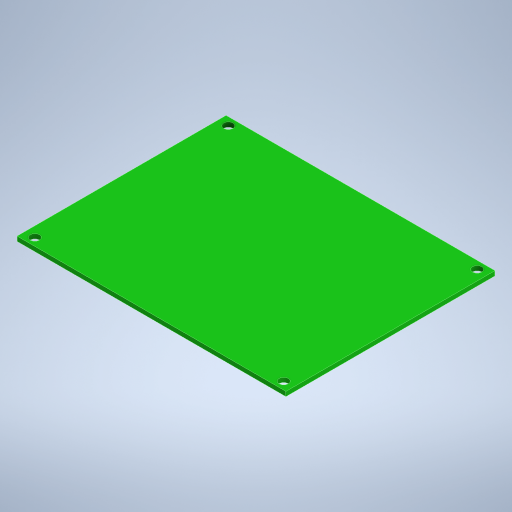
# Autodesk Inventor part: PCB
Saved by Autodesk Inventor 2024 (Build 280153000, 153)
## iProperties
Created: 2023-10-18
Part Number: PCB
Material: Generic
Document SubType Name: Modeling
Designer: CJ110
Density: 1 g/cm^3
Appearance: Default
Author: CJ110
Autodesk Inventor part; units mm, degrees
ref_plane "YZ Plane" through (0, 0, 0) normal (1, 0, 0) x (0, 1, 0)
ref_plane "XZ Plane" through (0, 0, 0) normal (0, 1, 0) x (-1, 0, 0)
ref_plane "XY Plane" through (0, 0, 0) normal (0, 0, 1) x (1, 0, 0)
sketch "Sketch1" plane through (0, 0, 0) normal (0, 1, 0) x (-1, 0, 0)
  line L0 (0, 0) -> (90.17, 0)
  line L1 (90.17, 0) -> (90.17, 70.104)
  line L2 (90.17, 70.104) -> (0, 70.104)
  line L3 (0, 70.104) -> (0, 0)
  dimension "PCB_Length" = 90.17
  dimension "PCB_Width" = 70.104
  constraints: 8 end point, 2 parallel, 1 horizontal, 1 perpendicular
  measures "PCB_Length" distance of L2.end L1.end
  measures "PCB_Width" distance of L0.end L1.end
extrude "Extrusion1" add sketch "Sketch1" along normal blind 1.524
sketch "Sketch2" plane through (0, 1.524, 0) normal (0, 1, 0) x (1, 0, 0)
  circle A0 centre (-3.3655, -2.6035) radius 1.5875
  circle A1 centre (-86.8045, -2.6035) radius 1.5875
  circle A2 centre (-86.8045, -67.5005) radius 1.5875
  circle A3 centre (-3.3655, -67.5005) radius 1.5875
  line L0 (-90.17, -70.104) -> (0, -70.104) projected
  line L1 (0, -70.104) -> (0, 0) projected
  line L2 (0, 0) -> (-90.17, 0) projected
  line L3 (-90.17, 0) -> (-90.17, -70.104) projected
  point P0 (-3.3655, -69.088)
  point P1 (-1.778, -67.5005)
  point P2 (-3.3655, -1.016)
  point P3 (-1.778, -2.6035)
  point P4 (-86.8045, -1.016)
  point P5 (-88.392, -2.6035)
  point P6 (-86.8045, -69.088)
  point P7 (-88.392, -67.5005)
  dimension "d4" = 3.175
  dimension "d5" = 1.016
  dimension "d6" = 1.778
  dimension "d7" = 1.016
  dimension "d8" = 1.778
  dimension "d9" = 1.016
  dimension "d10" = 1.778
  dimension "d11" = 1.016
  dimension "d12" = 1.778
  constraints: 8 point on circle, 4 centre point, 4 horizontal alignment, 4 vertical alignment, 3 equal radius
  measures "d4" diameter of A3
  measures "d5" distance from line of L0 A3.start
  measures "d6" distance from line of L1 A3.end
  measures "d7" distance from line of L2 A0.start
  measures "d8" distance from line of L1 A0.end
  measures "d9" distance from line of L0 A2.start
  measures "d10" distance from line of L3 A2.end
  measures "d11" distance from line of L2 A1.start
  measures "d12" distance from line of L3 A1.end
extrude "Extrusion2" cut sketch "Sketch2" against normal through all contours A0 | A1 | A2 | A3
body "Solid1"
